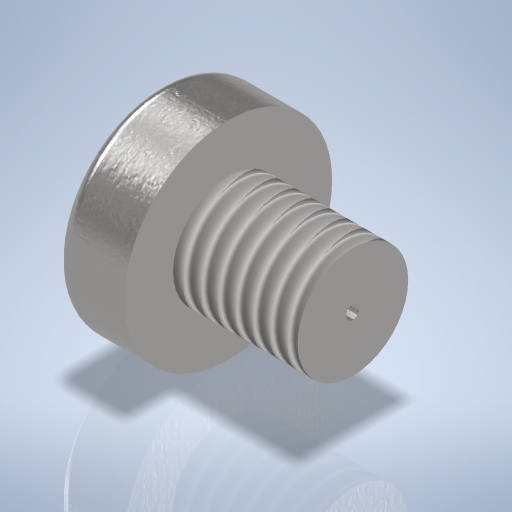
# Autodesk Inventor part: 1 part 4
Saved by Autodesk Inventor 2024 (Build 280153000, 153)
## iProperties
Created: 2024-07-24
Part Number: 1 part 4
Material: Stahl, galvanisiert
Document SubType Name: Modeling
Designer: ffogue
Density: 7.85 g/cm^3
Appearance: Galvanisiert
Author: ffogue
Autodesk Inventor part; units mm, degrees
ref_plane "YZ Plane" through (0, 0, 0) normal (1, 0, 0) x (0, 1, 0)
ref_plane "XZ Plane" through (0, 0, 0) normal (0, 1, 0) x (-1, 0, 0)
ref_plane "XY Plane" through (0, 0, 0) normal (0, 0, 1) x (1, 0, 0)
sketch "Skizze1" plane through (0, 0, 0) normal (0, 0, 1) x (1, 0, 0)
  line L0 (0, 0) -> (0, 7.5)
  line L1 (0, 7.5) -> (5, 7.5)
  line L2 (5, 7.5) -> (5, 4)
  line L3 (5, 4) -> (14, 4)
  line L4 (14, 4) -> (14, 0)
  line L5 (14, 0) -> (0, 0)
  dimension "d0" = 15
  dimension "d1" = 9
  dimension "d2" = 5
  dimension "d3" = 8
  constraints: 12 end point, 5 perpendicular, 1 vertical
  measures "d0" diameter of L1 L5
  measures "d1" distance of L2.end L3.end
  measures "d2" distance of L0.end L1.end
  measures "d3" diameter of L3 L5
revolve "Umdrehung1" add sketch "Skizze1" angle 360 about axis through (14, 0, 0) along (-1, 0, 0)
thread "Gewinde1" size "M8x1.25" class "6g" standard "ISO Metric profile" length 11
sketch "Skizze2" plane through (0, 0, 0) normal (-1, 0, 0) x (0, 0, 1)
  circle A0 centre (0, 0) radius 7.5 projected
  point P0 (0, 0)
  constraints: 1 coincident
hole "Bohrung1" at (0, 0, 0) direction (1, 0, 0) diameter 1 depth 14
fillet "Rundung1" radius 1 1 edges at (0, -7.5, 0)
